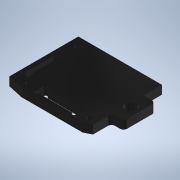
# Autodesk Inventor part: コックピット_サブフレーム_1_5_New
Saved by Autodesk Inventor 2020 (Build 240168000, 168)
## iProperties
Created: 2016-05-09
Part Number: コックピット_サブフレーム_1_5_New
Material: アセタール樹脂、黒
Document SubType Name: Modeling
Designer: hiroaki
Density: 1.425 g/cm^3
Appearance: 滑らか - 黒
Mass: 4.98887 g
Surface Area: 48.5671 cm^2
Volume: 3.50096 cm^3
Author: hiroaki
Autodesk Inventor part; units mm, degrees
ref_plane "YZ Plane" through (0, 0, 0) normal (1, 0, 0) x (0, 1, 0)
ref_plane "XZ Plane" through (0, 0, 0) normal (0, 1, 0) x (-1, 0, 0)
ref_plane "XY Plane" through (0, 0, 0) normal (0, 0, 1) x (1, 0, 0)
sketch "スケッチ1" plane through (0, 0, 0) normal (0, 0, 1) x (1, 0, 0)
  line L0 (-24.25, -20) -> (24.25, -20) construction
  line L1 (24.25, 20) -> (-24.25, 20)
  line L2 (-24.25, 20) -> (-24.25, -20)
  line L3 (-24.25, -20) -> (24.25, 20) construction
  line L4 (24.25, -20) -> (-24.25, 20) construction
  circle A0 centre (-15.25, -17.5) radius 1.55
  circle A1 centre (20.25, -17.5) radius 1.55
  line L5 (-9.25, -15) -> (14.25, -15) construction
  line L6 (14.25, -15) -> (14.25, -20) construction
  line L7 (14.25, -20) -> (-9.25, -20) construction
  line L8 (-9.25, -20) -> (-9.25, -15) construction
  line L9 (-24.25, -20) -> (-15.25, -22)
  line L10 (-15.25, -22) -> (20.25, -22)
  line L11 (20.25, -22) -> (24.25, -20)
  line L12 (14.3, -14.95) -> (-9.3, -14.95)
  line L13 (-9.3, -14.95) -> (-9.3, -20.05)
  line L14 (-9.3, -20.05) -> (14.3, -20.05)
  line L15 (14.3, -20.05) -> (14.3, -14.95)
  circle A2 centre (-8.25, -14.95) radius 1.05
  circle A3 centre (-8.25, -20.05) radius 1.05
  circle A4 centre (13.25, -14.95) radius 1.05
  circle A5 centre (13.25, -20.05) radius 1.05
  circle A6 centre (-19.25, 15) radius 1.55
  line L16 (-21.8, 5.05) -> (-19.2, 5.05)
  line L17 (-19.2, 5.05) -> (-19.2, -15.05)
  line L18 (-19.2, -15.05) -> (-21.8, -15.05)
  line L19 (-21.8, -15.05) -> (-21.8, 5.05)
  line L20 (-19.25, 5) -> (-21.75, 5) construction
  line L21 (-21.75, 5) -> (-21.75, -15) construction
  line L22 (-21.75, -15) -> (-19.25, -15) construction
  line L23 (-19.25, -15) -> (-19.25, 5) construction
  line L24 (2.5, -14.95) -> (2.5, -20.05) construction
  circle A7 centre (-21.8, 4) radius 1.05
  circle A8 centre (-19.2, 4) radius 1.05
  circle A9 centre (-21.8, -14) radius 1.05
  circle A10 centre (-19.2, -14) radius 1.05
  line L25 (24.25, 9.25) -> (31.25, 9.25)
  line L26 (31.25, 9.25) -> (31.25, -9.25)
  line L27 (31.25, -9.25) -> (24.25, -9.25)
  circle A11 centre (26.25, 0) radius 3.25
  line L28 (24.25, -20) -> (24.25, -9.25)
  line L29 (24.25, 9.25) -> (24.25, 20)
  point P0 (0, 0)
  point P1 (-9.25, -17.5)
  point P2 (12.2, -20.05)
  point P3 (-7.2, -20.05)
  point P4 (-7.2, -14.95)
  point P5 (12.2, -14.95)
  point P6 (-21.8, -12.95)
  point P7 (-21.8, 2.95)
  point P8 (-19.2, 2.95)
  point P9 (-19.2, -12.95)
  dimension "d10" = 2.1
  dimension "d26" = 2.1
  dimension "d0" = 5
  dimension "d3" = 3.1
  dimension "d4" = 35.5
  dimension "d5" = 2
  dimension "d7" = 40
  dimension "d8" = 23.5
  dimension "d9" = 0.05
  dimension "d11" = 3.1
  dimension "d12" = 5
  dimension "d13" = 5
  dimension "d14" = 0.05
  dimension "d15" = 17.75
  dimension "d16" = 48.5
  dimension "d20" = 2.5
  dimension "d21" = 2.5
  dimension "d22" = 5
  dimension "d23" = 15
  dimension "d27" = 25
  dimension "d58" = 6.5
  dimension "d60" = 9.25
  dimension "d61" = 18.5
  dimension "d62" = 20
  dimension "d65" = 2
  dimension "d66" = 5
  constraints: 60 end point, 12 parallel, 8 point on line, 7 perpendicular, 5 midpoint, 4 centre point, 4 horizontal, 2 horizontal alignment, 2 vertical alignment, 1 coincident, 1 collinear, 1 equal radius, 30 other
  measures "d0" distance of L7.end L5.start
  measures "d3" diameter of A0
  measures "d4" distance of A1.centre A0.centre
  measures "d5" distance between parallel lines of L10 L0
  measures "d7" distance of L0.end L1.start
  measures "d8" distance of L5.start L5.end
  measures "d9" distance between parallel lines of L12 L5
  measures "d11" diameter of A6
  measures "d12" distance from line of L2 A6.centre
  measures "d13" distance from line of L1 A6.centre
  measures "d14" distance between parallel lines of L16 L20
  measures "d15" distance from line of A0.centre L24
  measures "d16" distance of L1.start L1.end
  measures "d20" distance of L20.start L20.end
  measures "d21" distance between parallel lines of L21 L2
  measures "d22" distance between parallel lines of L22 L0
  measures "d23" distance between parallel lines of L1 L20
  measures "d27" distance between parallel lines of L20 L0
  measures "d58" diameter of A11
  measures "d60" distance from line of L25 A11.centre
  measures "d61" distance between parallel lines of L27 L25
  measures "d62" distance from line of A11.centre L1
  measures "d65" distance from line of L29 A11.centre
  measures "d66" distance from line of A11.centre L26
extrude "押し出し1" add sketch "スケッチ1" along normal blind 5
sketch "スケッチ2" plane through (0, 0, 0) normal (0, 0, -1) x (-1, 0, 0)
  line L0 (-14.3, -20.05) -> (-14.3, -14.95) projected
  line L1 (-12.2, -14.95) -> (7.2, -14.95) projected
  line L2 (-24.25, 20) -> (24.25, 20) projected
  line L3 (-24.25, -20) -> (-24.25, 20) projected
  line L4 (21.8, -15.05) -> (19.2, -15.05) projected
  line L5 (19.2, -12.95) -> (19.2, 2.95) projected
  line L6 (19.2, 5.05) -> (21.8, 5.05) projected
  line L7 (-20.25, 16) -> (16.25, 16)
  line L8 (16.25, 16) -> (16.25, -11)
  line L9 (16.25, -11) -> (-20.25, -11)
  line L10 (-20.25, -11) -> (-20.25, -5.9161)
  line L11 (-20.25, 16) -> (-20.25, 5.9161)
  line L12 (19.25, 5.05) -> (19.25, -15.05) construction
  line L13 (19.2, -15.05) -> (21.8, -15.05) projected
  line L14 (-14.3, -15) -> (9.3, -15) construction
  line L15 (9.3, -20.05) -> (9.3, -14.95) projected
  line L16 (-20.25, 5.9161) -> (-20.25, -5.9161)
  point P0 (0, 0)
  dimension "d29" = 4
  dimension "d30" = 4
  dimension "d31" = 0.05
  dimension "d32" = 3
  dimension "d33" = 0.05
  dimension "d34" = 4
  constraints: 16 end point, 4 point on line, 3 perpendicular, 3 vertical, 2 horizontal, 1 vertical alignment
  measures "d29" distance between parallel lines of L3 L11
  measures "d30" distance between parallel lines of L2 L7
  measures "d31" distance between parallel lines of L12 L5
  measures "d32" distance between parallel lines of L8 L12
  measures "d33" distance between parallel lines of L1 L14
  measures "d34" distance between parallel lines of L14 L9
sketch "スケッチ3" plane through (0, 0, 0) normal (0, 0, -1) x (-1, 0, 0)
  circle A0 centre (15.25, -17.5) radius 1.55 projected
  circle A1 centre (15.25, -17.5) radius 3
  circle A2 centre (19.25, 15) radius 1.55 projected
  circle A3 centre (19.25, 15) radius 3
  circle A4 centre (-20.25, -17.5) radius 3
  point P0 (0, 0)
  dimension "d38" = 6
  dimension "d39" = 6
  dimension "d40" = 6
  constraints: 3 centre point, 2 coincident
  measures "d38" diameter of A1
  measures "d39" diameter of A3
  measures "d40" diameter of A4
extrude "押し出し3" cut sketch "スケッチ3" against normal blind 3.5 contours A1 | A4
extrude "押し出し5" cut sketch "スケッチ2" against normal blind 3
fillet "フィレット4" radius 2 4 edges at (20.25, -11, 1.5) (20.25, 16, 1.5) (-16.25, 16, 1.5) (-16.25, -11, 1.5)
fillet "フィレット5" radius 2 3 edges at (24.25, -9.25, 2.5) (31.25, -9.25, 2.5) (31.25, 9.25, 2.5)
equation "\"d13\" = d12"
equation "\"d15\" = 0.5 * d4"
equation "\"d60\" = 0.5 * d61"
